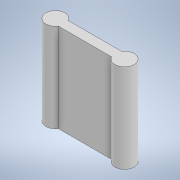
# Autodesk Inventor part: 7
Saved by Autodesk Inventor 2020 (Build 240168000, 168)
## iProperties
Created: 2019-08-08
Part Number: 7
Material: Generic
Document SubType Name: Modeling
Designer: Nicolas
Density: 1 g/cm^3
Appearance: Default
Author: Nicolas
Autodesk Inventor part; units mm, degrees
ref_plane "YZ Plane" through (0, 0, 0) normal (1, 0, 0) x (0, 1, 0)
ref_plane "XZ Plane" through (0, 0, 0) normal (0, 1, 0) x (-1, 0, 0)
ref_plane "XY Plane" through (0, 0, 0) normal (0, 0, 1) x (1, 0, 0)
sketch "Sketch1" plane through (0, 0, 0) normal (0, 1, 0) x (-1, 0, 0)
  circle A0 centre (-6.5431, 0.4696) radius 2.1574
  line L0 (-4.6497, 1.5037) -> (7.3503, 1.5037)
  line L1 (7.272, -0.6963) -> (-4.728, -0.6963)
  circle A1 centre (9.1656, 0.3377) radius 2.1575
  point P0 (0, 0)
  point P1 (0, 0)
  point P2 (0, 0)
  dimension "d0" = 4.3147
  dimension "d2" = 12
  dimension "d3" = 4.315
  dimension "d8" = 2.2
  dimension "d9" = 12
  constraints: 4 end point, 4 point on circle, 2 centre point, 2 horizontal
  measures "d0" diameter of A0
  measures "d2" distance of L0.start L0.end
  measures "d3" diameter of A1
  measures "d8" distance between parallel lines of L1 L0
  measures "d9" distance of L1.start L1.end
extrude "Extrusion1" add sketch "Sketch1" along normal blind 20
body "Solid1"
